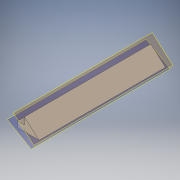
# Autodesk Inventor part: Ramp version 2 {needs editing}
Saved by Autodesk Inventor 2019 (Build 230136000, 136)
## iProperties
Created: 2019-01-24
Part Number: Ramp version 2 {needs editing}
Material: Generic
Document SubType Name: Modeling
Designer: Ashley
Density: 1 g/cm^3
Appearance: Default
Author: Ashley
Autodesk Inventor part; units mm, degrees
ref_plane "YZ Plane" through (0, 0, 0) normal (1, 0, 0) x (0, 1, 0)
ref_plane "XZ Plane" through (0, 0, 0) normal (0, 1, 0) x (-1, 0, 0)
ref_plane "XY Plane" through (0, 0, 0) normal (0, 0, 1) x (1, 0, 0)
sketch "Sketch1" plane through (0, 0, 0) normal (0, 1, 0) x (-1, 0, 0)
  line L0 (12.2947, 115.8176) -> (-13.1053, 115.8176)
  line L1 (-13.1053, 115.8176) -> (-13.1053, -31.6824)
  line L2 (-13.1053, -31.6824) -> (12.2947, -31.6824)
  line L3 (12.2947, -31.6824) -> (12.2947, 115.8176)
  point P0 (0, 0)
  dimension "d0" = 25.4
  dimension "d1" = 147.5
  constraints: 8 end point, 2 parallel, 1 horizontal, 1 perpendicular
  measures "d0" distance between parallel lines of L1 L3
  measures "d1" distance between parallel lines of L0 L2
extrude "Extrusion1" add sketch "Sketch1" along normal blind 15
sketch "Sketch2" plane through (-12.2947, 0, 115.8176) normal (0, 0, 1) x (1, 0, 0)
  line L0 (0, 15) -> (8, 15)
  line L1 (8, 15) -> (8, 7)
  line L2 (8, 7) -> (0, 7)
  line L3 (0, 7) -> (0, 15)
  point P0 (12.2947, 0)
  dimension "d13" = 8
  constraints: 8 end point, 2 parallel, 1 horizontal, 1 perpendicular
  measures "d13" distance between parallel lines of L2 L0
extrude "Extrusion2" cut sketch "Sketch2" against normal through all
ref_plane "Work Plane1" through (-4.2947, 15, 78.9426) normal (0.6561, 0.7547, 0) x (0, 0, 1)
sketch "Sketch3" plane through (-4.2947, 15, 78.9426) normal (0.6561, 0.7547, 0) x (0, 0, 1)
  line L0 (36.875, 0) -> (36.875, 13.1319) construction
  line L1 (-110.625, 22.9728) -> (-110.625, 3.8032) construction
  line L2 (36.875, 0) -> (-110.625, 0)
  line L3 (-110.625, 0) -> (-110.625, 22.9728)
  line L4 (-110.625, 22.9728) -> (36.875, 22.9728)
  line L5 (36.875, 22.9728) -> (36.875, 0)
  point P0 (-78.9426, 13.0821)
  constraints: 8 end point, 2 parallel, 1 horizontal, 1 perpendicular
extrude "Extrusion3" add sketch "Sketch3" along normal blind 15
sketch "Sketch4" plane through (5.5462, 26.3206, 78.9426) normal (0.6561, 0.7547, 0) x (0.7547, -0.6561, 0)
  line L0 (22.8638, 110.625) -> (22.8638, -36.875) construction
  line L1 (0, -36.875) -> (22.8638, -36.875)
  line L2 (-1.723, -37.6113) -> (24.2555, -37.6113)
  line L3 (24.2555, -37.6113) -> (24.2555, 112.242)
  line L4 (24.2555, 112.242) -> (-1.723, 112.242)
  line L5 (-1.723, 112.242) -> (-1.723, -37.6113)
  constraints: 10 end point, 2 horizontal, 2 parallel, 1 perpendicular
extrude "Extrusion4" cut sketch "Sketch4" against normal blind 15
ref_plane "Work Plane2" through (-12.2947, 7, 42.0676) normal (-0.5, -0.866, 0) x (0, 0, -1)
sketch "Sketch5" plane through (-12.2947, 7, 42.0676) normal (-0.5, -0.866, 0) x (0, 0, -1)
  point P0 (42.0676, 14.1475)
body "Solid1"
